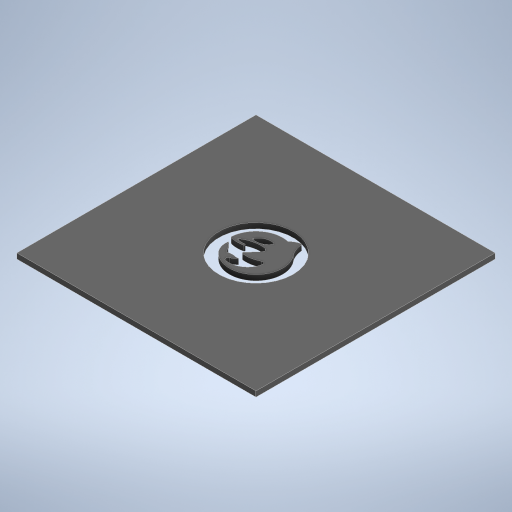
# Autodesk Inventor part: ROGO
Saved by Autodesk Inventor 2024.1 (Build 281209000, 209)
## iProperties
Created: 2025-01-20
Part Number: ROGO
Material: 一般
Document SubType Name: Modeling
Designer: hibik
Density: 1 g/cm^3
Appearance: 既定
Author: hibik
Autodesk Inventor part; units mm, degrees
ref_plane "YZ Plane" through (0, 0, 0) normal (1, 0, 0) x (0, 1, 0)
ref_plane "XZ Plane" through (0, 0, 0) normal (0, 1, 0) x (-1, 0, 0)
ref_plane "XY Plane" through (0, 0, 0) normal (0, 0, 1) x (1, 0, 0)
sketch "スケッチ1" plane through (0, 0, 0) normal (0, 1, 0) x (-1, 0, 0)
  circle A0 centre (0, 0) radius 10
  circle A1 centre (-15.3704, -12) radius 9.5
  circle A2 centre (-7.8, -3.3779) radius 8.5
  line L0 (10, -10) -> (-10, -10)
  line L1 (-10, -10) -> (-10, 10)
  line L2 (-10, 10) -> (10, 10)
  line L3 (10, 10) -> (10, -10)
  point P0 (-2.1842, -9.7585)
  point P1 (-7.8823, -6.1538)
  point P2 (-5.8766, -11.6574)
  dimension "d7" = 17
  dimension "d0" = 20
  dimension "d1" = 2
  dimension "d2" = 19
  dimension "d8" = 7.8
  constraints: 8 end point, 5 tangent, 2 centre point, 2 parallel, 1 coincident, 1 horizontal, 1 perpendicular, 3 other
  measures "d0" diameter of A0
  measures "d1" distance from line of A1.centre L0
  measures "d2" diameter of A1
  measures "d8" horizontal distance of point (0, 0) point (-7.8, -3.378)
extrude "押し出し1" add sketch "スケッチ1" along normal blind 2 contours A0 A2 | A2 A0 | A2 L0 A1 A0 | A2 A1 L0
fillet "フィレット1" radius 0.4 1 edges at (5.8766, 1, -11.6574)
sketch "スケッチ2" plane through (0, 2, 0) normal (0, 1, 0) x (1, 0, 0)
  arc A0 (2.1842, 9.7585) -> (7.8823, 6.1538) centre (0, 0) ccw projected
  circle A1 centre (0, 0) radius 10
  line L0 (10, 10) -> (10, -15.213)
  circle A2 centre (-1.5, -8.1667) radius 11.5
  circle A3 centre (-1, -2) radius 6
  line L1 (-1, -2) -> (-9.9915, -0.4114)
  point P0 (-4.3575, 2.9727)
  point P1 (3.1147, 2.3668)
  point P2 (-6.9085, -0.9561)
  dimension "d12" = 23
  dimension "d13" = 8.1667
  dimension "d14" = 12
  dimension "d15" = 2
  dimension "d16" = 1
  constraints: 4 end point, 3 vertical, 2 coincident, 1 centre point, 7 other
  measures "d13" vertical distance of point (0, 0) point (-1.5, -8.167)
  measures "d14" diameter of A3
  measures "d15" vertical distance of point (0, 0) L1.start
  measures "d16" horizontal distance of point (0, 0) L1.start
extrude "押し出し2" cut sketch "スケッチ2" against normal through all contours A2 A3 L1 | A2 A3 picked at (-0.8922, -0.5087)
sketch "スケッチ3" plane through (0, 2, 0) normal (0, 1, 0) x (1, 0, 0)
  arc A0 (2.1842, 9.7585) -> (7.8823, 6.1538) centre (0, 0) ccw projected
  circle A1 centre (-9.4656, 0.8083) radius 0.5
  arc A2 (3.1147, 2.3668) -> (-9.9915, -0.4114) centre (-1.5, -8.1667) ccw projected
  circle A3 centre (-7.065, 10) radius 10
  line L0 (-23.9276, 0) -> (19.7195, 0) projected
  circle A4 centre (-5.9539, 10.7692) radius 10
  circle A5 centre (-4.9754, 0.5217) radius 0.2941
  circle A6 centre (-7.7516, 1.1864) radius 0.25
  point P0 (-5.0034, 0.8145)
  point P1 (-7.7977, 0.9407)
  point P2 (-7.8905, 1.3942)
  point P3 (-9.3266, 0.2591)
  point P4 (-4.9121, 0.2345)
  point P5 (-9.5919, 0.3245)
  point P6 (-9.9637, 0.8508)
  dimension "d19" = 1
  dimension "d20" = 20
  dimension "d22" = 1.1111
  dimension "d23" = 0.7692
  dimension "d24" = 0.5882
  dimension "d25" = 20
  dimension "d26" = 0.5
  constraints: 8 tangent, 5 centre point
  measures "d19" diameter of A1
  measures "d20" diameter of A3
  measures "d22" horizontal distance of A4.centre A3.centre
  measures "d23" vertical distance of A3.centre A4.centre
  measures "d24" diameter of A5
  measures "d25" diameter of A4
  measures "d26" diameter of A6
extrude "押し出し3" add sketch "スケッチ3" against normal up to surface (2 mm away) contours A5 | A4 A5 A3 A2 | A2 A6 A4
extrude "押し出し4" cut sketch "スケッチ3" against normal through all contours A1 A3 A0 | A3 A2 L0 A0 | L0 A2 A0 picked at (-9.7757, -0.045)
sketch "スケッチ4" plane through (0, 2, 0) normal (0, 1, 0) x (1, 0, 0)
  circle A0 centre (-23, 20) radius 30
  circle A1 centre (-1, 7.1429) radius 10
  arc A2 (-9.9915, -0.4114) -> (7.8823, 6.1538) centre (0, 0) ccw projected
  line L0 (20, -10) -> (-13, -10)
  circle A3 centre (-2.1753, -2.2842) radius 0.5
  circle A4 centre (4.1522, -2.3869) radius 0.8333
  arc A5 (-6.9085, -0.9561) -> (3.1147, 2.3668) centre (-1, -2) ccw projected
  arc A6 (3.1147, 2.3668) -> (-7.8905, 1.3942) centre (-1.5, -8.1667) ccw projected
  circle A7 centre (0.2271, 2.3592) radius 0.8333
  point P0 (-2.2372, -2.7803)
  point P1 (3.7558, -1.6538)
  point P2 (4.9832, -2.4493)
  point P3 (0.362, 3.1816)
  point P4 (0.8907, 1.8552)
  point P5 (-2.5167, -1.9188)
  dimension "d31" = 60
  dimension "d32" = 20
  dimension "d33" = 1
  dimension "d34" = 7.1429
  dimension "d36" = 23
  dimension "d37" = 1
  dimension "d38" = 1.6667
  constraints: 8 tangent, 5 centre point, 2 end point, 1 equal radius, 1 horizontal
  measures "d31" diameter of A0
  measures "d32" diameter of A1
  measures "d33" horizontal distance of point (0, 0) A1.centre
  measures "d34" vertical distance of point (0, 0) A1.centre
  measures "d36" horizontal distance of point (0, 0) A0.centre
  measures "d37" diameter of A3
  measures "d38" diameter of A7
extrude "押し出し5" add sketch "スケッチ4" against normal up to surface (2 mm away) contours A6 A5 A1 A3 A0 | A0 A7 A6 | A4 A1 A5 | A3
sketch "スケッチ5" plane through (0, 2, 0) normal (0, 1, 0) x (1, 0, 0)
  circle A0 centre (-2.4495, -2.5) radius 6.5
  arc A1 (-9.9915, -0.4114) -> (7.8823, 6.1538) centre (0, 0) ccw projected
  line L0 (-6.9085, -0.9561) -> (-9.9915, -0.4114) projected
  circle A2 centre (-7.0815, -1.1194) radius 1.6667
  circle A3 centre (-11.0471, -6.4783) radius 5
  arc A4 (-6.9085, -0.9561) -> (4.9832, -2.4493) centre (-1, -2) ccw projected
  circle A5 centre (-4, -9.9026) radius 5
  circle A6 centre (-5.8364, -4.7182) radius 0.5
  circle A7 centre (-2.2376, -3.4731) radius 1.6667
  circle A8 centre (-6.1854, -0.6847) radius 6.5
  circle A9 centre (-4.5455, -7.7993) radius 0.8012
  line L1 (-7.0815, -1.1194) -> (-5.8364, -4.7182)
  line L2 (-5.8364, -4.7182) -> (-2.2376, -3.4731)
  line L3 (-5.8364, -4.7182) -> (-2.4495, -2.5)
  line L4 (-5.8364, -4.7182) -> (-6.1854, -0.6847)
  circle A10 centre (-2, -1.1725) radius 7.0989
  circle A11 centre (-3.2111, -7.3526) radius 0.8012
  point P0 (-8.6787, -0.6434)
  point P1 (-4.4093, -6.9373)
  point P2 (-0.8762, -4.4347)
  point P3 (-2.6782, -5.0805)
  point P4 (-5.6694, -5.1895)
  point P5 (-6.1181, -5.1313)
  point P6 (-4.8401, -8.5444)
  point P7 (0.6968, -8.1878)
  point P8 (0.5364, -7.8)
  point P9 (-4.1933, -7.0796)
  point P10 (-6.4802, -4.4427)
  point P11 (-6.3101, -4.8782)
  point P12 (-7.6299, -6.4641)
  point P13 (-7.6138, -6.4471)
  point P14 (-8.9262, -1.9505)
  point P15 (-4.7254, -7.0186)
  point P16 (2.1141, -7.1286)
  point P17 (-8.0729, -2.4592)
  point P18 (-3.9972, -7.1977)
  point P19 (-3.5375, -6.6209)
  point P20 (-4.0654, -7.1578)
  point P21 (0.5607, -7.7935)
  point P22 (-3.3652, -8.1389)
  point P23 (-7.0094, -7.1322)
  point P24 (-7.0093, -7.1322)
  dimension "d41" = 13
  dimension "d43" = 3.3333
  dimension "d42" = 2.5
  dimension "d44" = 10
  dimension "d45" = 10
  dimension "d46" = 1
  dimension "d47" = 3.3333
  dimension "d50" = 4
  dimension "d53" = 4.5454
  dimension "d54" = 90
  dimension "d59" = 2
  constraints: 8 centre point, 8 end point, 8 tangent, 2 equal length, 2 point on circle, 1 equal radius, 1 point on line, 10 other
  measures "d42" vertical distance of point (0, 0) L3.end
  measures "d44" diameter of A3
  measures "d45" diameter of A5
  measures "d46" diameter of A6
  measures "d47" diameter of A7
  measures "d50" horizontal distance of point (0, 0) A5.centre
  measures "d53" horizontal distance of point (0, 0) A9.centre
  measures "d54" angle of L2 L1
  measures "d59" horizontal distance of point (0, 0) A10.centre
extrude "押し出し6" add sketch "スケッチ5" against normal up to surface (2 mm away) contours A10 A4 A0 | A0 A4 A10 | A8 A5 A7 | A5 A8 A4 | A5 A4 A6 | A11 A4 A9 A8 | A4 A9
extrude "押し出し7" cut sketch "スケッチ5" against normal through all contours A0 A3 A10 L0 | L0 A4 A2 | A10 A5 A4 | A0 A10 A3 | A10 A3 A1 L0 | A2 A4 A3 | A5 A10 A11 A4 | A0 A5 A1 A3 A10 | A4 A6 A3 | A11 A9 A4 | A6 A4 | A11 A9 picked at (-3.3615, -7.7258)
sketch "スケッチ6" plane through (0, 2, 0) normal (0, 1, 0) x (1, 0, 0)
  arc A0 (-7.6299, -6.4641) -> (7.8823, 6.1538) centre (0, 0) ccw projected
  arc A1 (-8.6787, -0.6434) -> (-7.6138, -6.4471) centre (-2.4495, -2.5) ccw projected
  circle A2 centre (-2.4495, -2.5) radius 6.5
  arc A3 (-7.6138, -6.4471) -> (-7.6299, -6.4641) centre (-4, -9.9026) ccw projected
  point P0 (-7.6138, -6.4471)
  point P1 (-6.9985, -7.1429)
  constraints: 2 concentric, 1 centre point
extrude "押し出し8" cut sketch "スケッチ6" against normal through all contours A3 A2 A0
fillet "フィレット2" radius 0.1 2 edges at (-8.6787, 1, 0.6434) (-0.8762, 1, 4.4347)
sketch "スケッチ7" plane through (0, 2, 0) normal (0, 1, 0) x (1, 0, 0)
  arc A0 (2.1842, 9.7585) -> (-9.9637, 0.8508) centre (0, 0) ccw projected
  circle A1 centre (0, 0) radius 10
  circle A2 centre (-3.8462, 8.6957) radius 5
  circle A3 centre (-1, 1.6667) radius 5
  circle A4 centre (-4.9447, 4.1601) radius 0.3333
  circle A5 centre (0.0985, 6.2022) radius 0.3333
  point P0 (0.598, 6.4044)
  point P1 (-5.4441, 3.9579)
  point P2 (0.177, 6.5262)
  point P3 (-5.2264, 4.3382)
  point P4 (-5.0231, 3.8362)
  point P5 (0.3803, 6.0241)
  dimension "d63" = 10
  dimension "d64" = 1.6667
  dimension "d65" = 1
  dimension "d66" = 3.8462
  dimension "d67" = 8.6957
  dimension "d70" = 0.6667
  constraints: 5 centre point, 4 tangent, 3 equal radius, 1 concentric
  measures "d63" diameter of A3
  measures "d64" vertical distance of point (0, 0) A3.centre
  measures "d65" horizontal distance of point (0, 0) A3.centre
  measures "d66" horizontal distance of point (0, 0) A2.centre
  measures "d67" vertical distance of point (0, 0) A2.centre
  measures "d70" diameter of A4
extrude "押し出し9" cut sketch "スケッチ7" against normal through all contours A4 A3 A5 A2 | A4 | A5
sketch "スケッチ8" plane through (0, 2, 0) normal (0, 1, 0) x (1, 0, 0)
  circle A0 centre (0, 0) radius 14
  line L0 (-45, -45) -> (45, -45)
  line L1 (45, -45) -> (45, 45)
  line L2 (45, 45) -> (-45, 45)
  line L3 (-45, 45) -> (-45, -45)
  line L4 (-45, -45) -> (45, 45) construction
  line L5 (45, -45) -> (-45, 45) construction
  dimension "d71" = 28
  dimension "d72" = 90
  constraints: 12 end point, 2 midpoint, 2 parallel, 2 perpendicular, 1 centre point, 1 coincident, 1 horizontal
  measures "d71" diameter of A0
  measures "d72" distance of L0.end L1.end
extrude "押し出し10" add sketch "スケッチ8" against normal up to surface (2 mm away)
equation "\"d7\" = 1.7 * R"
equation "\"d0\" = 2 * R"
equation "\"d1\" = 0.2 * R"
equation "\"d2\" = 1.9 * R"
equation "\"d8\" = 0.78 * R"
equation "\"d11\" = 0.04 * R"
equation "\"d12\" = 2.3 * R"
equation "\"d13\" = 0.5 * d12 - 0.333333 * R"
equation "\"d14\" = 1.2 * R"
equation "\"d15\" = 0.2 * R"
equation "\"d16\" = 0.1 * R"
equation "\"d19\" = 0.1 * R"
equation "\"d20\" = 2 * R"
equation "\"d22\" = 0.111111 * R"
equation "\"d23\" = 0.0769231 * R"
equation "\"d24\" = 0.0588235 * R"
equation "\"d25\" = 2 * R"
equation "\"d26\" = 0.05 * R"
equation "\"d31\" = 6 * R"
equation "\"d32\" = 2 * R"
equation "\"d33\" = 0.1 * R"
equation "\"d34\" = 0.714286 * R"
equation "\"d36\" = 2.3 * R"
equation "\"d38\" = 0.166667 * R"
equation "\"d41\" = 1.3 * R"
equation "\"d43\" = 0.333333 * R"
equation "\"d42\" = 0.25 * R"
equation "\"d44\" = R"
equation "\"d45\" = R"
equation "\"d46\" = 0.1 * R"
equation "\"d47\" = 0.333333 * R"
equation "\"d50\" = 0.4 * R"
equation "\"d53\" = 0.454545 * R"
equation "\"R\" = 10"
